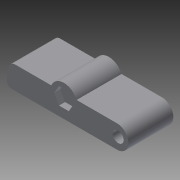
# Autodesk Inventor part: FelixOriginalBearingHolder
Saved by Autodesk Inventor 2015 SP1 (Build 190203100, 203)
## iProperties
Created: 2014-12-14
Part Number: FelixOriginalBearingHolder
Material: Generic
Document SubType Name: Modeling
Designer: Jack
Density: 1 g/cm^3
Appearance: Default
Author: Jack
Autodesk Inventor part; units mm, degrees
ref_plane "YZ Plane" through (0, 0, 0) normal (1, 0, 0) x (0, 1, 0)
ref_plane "XZ Plane" through (0, 0, 0) normal (0, 1, 0) x (-1, 0, 0)
ref_plane "XY Plane" through (0, 0, 0) normal (0, 0, 1) x (1, 0, 0)
sketch "Sketch1" plane through (0, 0, 0) normal (0, 0, 1) x (1, 0, 0)
  line L0 (0, 0) -> (1.4521, 9.38)
  line L1 (1.4521, 9.38) -> (50.35, 9.38)
  line L2 (50.35, 9.38) -> (50.35, 0)
  line L3 (50.35, 0) -> (0, 0)
  dimension "d7" = 81.2
  dimension "d8" = 50.35
  dimension "d9" = 9.38
  constraints: 8 end point, 2 perpendicular, 1 horizontal
  measures "d7" angle of L3 L0
  measures "d8" distance of L2.end L0.start
  measures "d9" distance of L1.end L2.end
extrude "Extrusion1" add sketch "Sketch1" along normal blind 18.5
fillet "Fillet1" radius 2.85 1 edges at (1.4521, 9.38, 9.25)
fillet "Fillet2" radius 1.85 1 edges at (0, 0, 9.25)
sketch "Sketch3" plane through (0, 0, 18.5) normal (0, 0, 1) x (1, 0, 0)
  line L0 (2.1584, 0) -> (50.35, 0) projected
  line L1 (50.35, 0) -> (50.35, 9.38) projected
  circle A0 centre (46.18, 4.8) radius 2.25
  point P0 (0, 0)
  dimension "d13" = 4.5
  dimension "d14" = 4.8
  dimension "d15" = 4.17
  constraints: 1 centre point
  measures "d13" diameter of A0
  measures "d14" distance from line of L0 A0.centre
  measures "d15" distance from line of L1 A0.centre
extrude "Extrusion2" cut sketch "Sketch3" against normal up to next
fillet "Fillet3" radius 4.6 2 edges at (50.35, 9.38, 9.25) (50.35, 0, 9.25)
sketch "Sketch5" plane through (0, 0, 18.5) normal (0, 0, 1) x (1, 0, 0)
  line L0 (45.75, 9.38) -> (3.8948, 9.38) projected
  arc A0 (29.0413, 9.38) -> (18.6587, 9.38) centre (23.85, 7.28) ccw
  point P0 (50.35, 4.6)
  point P1 (0, 0)
  dimension "d24" = 11.2
  dimension "d25" = 2.1
  dimension "d26" = 26.5
  constraints: 2 point on circle, 2 point on line, 1 centre point
  measures "d24" diameter of A0
  measures "d25" distance from line of L0 A0.centre
  measures "d26" horizontal distance of point (50.35, 4.6) A0.centre
extrude "Extrusion4" add sketch "Sketch5" against normal up to surface (18.5 mm away)
sketch "Sketch6" plane through (0, 0, 18.5) normal (0, 0, 1) x (1, 0, 0)
  arc A0 (29.0413, 9.38) -> (18.6587, 9.38) centre (23.85, 7.28) ccw projected
  line L0 (27.8915, 7.28) -> (25.8707, 3.78)
  line L1 (25.8707, 3.78) -> (21.8293, 3.78)
  line L2 (21.8293, 3.78) -> (19.8085, 7.28)
  line L3 (19.8085, 7.28) -> (21.8293, 10.78)
  line L4 (21.8293, 10.78) -> (25.8707, 10.78)
  line L5 (25.8707, 10.78) -> (27.8915, 7.28)
  point P0 (0, 0)
  dimension "d29" = 7
  constraints: 12 end point, 1 coincident, 1 horizontal, 13 other
  measures "d29" distance between parallel lines of L1 L4
extrude "Extrusion5" cut sketch "Sketch6" against normal blind 2.5
body "Solid1"
